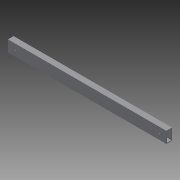
# Autodesk Inventor part: frame_wide
Saved by Autodesk Inventor 2015 SP1 (Build 190203100, 203)
## iProperties
Created: 2014-12-28
Part Number: frame_wide
Material: Generic
Document SubType Name: Modeling
Designer: Jarod
Density: 1 g/cm^3
Appearance: Default
Author: Jarod
Autodesk Inventor part; units mm, degrees
ref_plane "YZ Plane" through (0, 0, 0) normal (1, 0, 0) x (0, 1, 0)
ref_plane "XZ Plane" through (0, 0, 0) normal (0, 1, 0) x (-1, 0, 0)
ref_plane "XY Plane" through (0, 0, 0) normal (0, 0, 1) x (1, 0, 0)
sketch "Sketch1" plane through (0, 0, 0) normal (1, 0, 0) x (0, 1, 0)
  line L0 (0, 0) -> (50.8, 0)
  line L1 (50.8, 0) -> (50.8, -25.4)
  line L2 (50.8, -25.4) -> (0, -25.4)
  line L3 (0, -25.4) -> (0, 0)
  line L4 (3.175, -3.175) -> (47.625, -3.175)
  line L5 (47.625, -3.175) -> (47.625, -22.225)
  line L6 (47.625, -22.225) -> (3.175, -22.225)
  line L7 (3.175, -22.225) -> (3.175, -3.175)
  dimension "d0" = 50.8
  dimension "d1" = 25.4
  dimension "d2" = 44.45
  dimension "d3" = 19.05
  dimension "d4" = 3.175
  dimension "d5" = 3.175
  constraints: 16 end point, 4 parallel, 2 horizontal, 2 perpendicular
  measures "d0" distance of L1.end L2.end
  measures "d1" distance of L0.end L1.end
  measures "d2" distance of L5.end L6.end
  measures "d3" distance of L4.end L5.end
  measures "d4" distance between parallel lines of L3 L7
  measures "d5" distance between parallel lines of L0 L4
extrude "Extrusion1" add sketch "Sketch1" along normal blind 711.2
sketch "Sketch2" plane through (0, 0, 0) normal (0, 0, 1) x (1, 0, 0)
  line L0 (0, 0) -> (0, 50.8) projected
  line L1 (0, 0) -> (711.2, 0) projected
  line L2 (711.2, 50.8) -> (711.2, 0) projected
  line L3 (0, 50.8) -> (711.2, 50.8) projected
  point P0 (31.75, 25.4)
  point P1 (679.45, 25.4)
  dimension "d8" = 31.75
  dimension "d9" = 25.4
  dimension "d10" = 31.75
  dimension "d11" = 25.4
  measures "d8" distance from line of L0 point (31.75, 25.4)
  measures "d9" distance from line of L1 point (31.75, 25.4)
  measures "d10" distance from line of L2 point (679.45, 25.4)
  measures "d11" distance from line of L1 point (679.45, 25.4)
hole "Hole3" at (31.75, 25.4, 0) at (679.45, 25.4, 0) direction (0, 0, -1) diameter 6.35 end through all
sketch "Sketch3" plane through (0, 0, 0) normal (0, 0, 1) x (1, 0, 0)
  circle A0 centre (31.75, 25.4) radius 3.175 projected
  circle A1 centre (679.45, 25.4) radius 3.175 projected
  line L0 (0, 0) -> (0, 50.8) projected
  line L1 (0, 0) -> (711.2, 0) projected
  line L2 (711.2, 50.8) -> (711.2, 0) projected
  line L3 (0, 50.8) -> (711.2, 50.8) projected
  point P0 (95.25, 25.4)
  point P1 (615.95, 25.4)
  dimension "d37" = 95.25
  dimension "d38" = 25.4
  dimension "d39" = 25.4
  dimension "d40" = 95.25
  measures "d37" distance from line of L2 point (615.95, 25.4)
  measures "d38" distance from line of L1 point (615.95, 25.4)
  measures "d39" distance from line of L1 point (95.25, 25.4)
  measures "d40" distance from line of L0 point (95.25, 25.4)
hole "Hole4" at (95.25, 25.4, 0) at (615.95, 25.4, 0) direction (0, 0, -1) diameter 6.35 end through all
body "Solid1"
